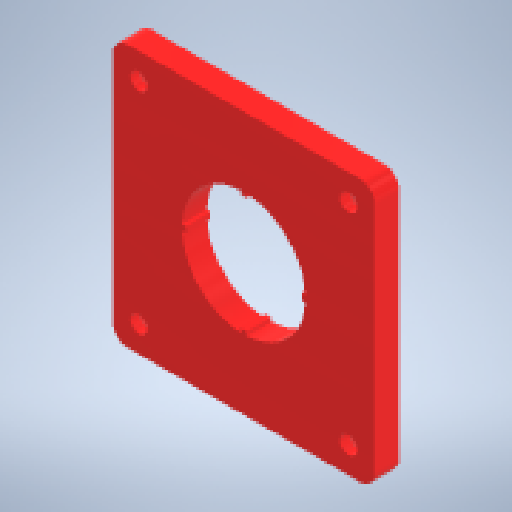
# Autodesk Inventor part: Parte1
Saved by Autodesk Inventor 2024 (Build 280153000, 153)
## iProperties
Created: 2023-12-16
Part Number: Parte1
Material: Generico
Document SubType Name: Modeling
Designer: cecca
Density: 1 g/cm^3
Appearance: Rosso chiaro
Author: cecca
Autodesk Inventor part; units mm, degrees
ref_plane "YZ Plane" through (0, 0, 0) normal (1, 0, 0) x (0, 1, 0)
ref_plane "XZ Plane" through (0, 0, 0) normal (0, 1, 0) x (-1, 0, 0)
ref_plane "XY Plane" through (0, 0, 0) normal (0, 0, 1) x (1, 0, 0)
sketch "Schizzo1" plane through (0, 0, 0) normal (0, 0, 1) x (1, 0, 0)
  line L0 (37.5, -42.5) -> (-37.5, -42.5)
  line L1 (-42.5, -37.5) -> (-42.5, 37.5)
  line L2 (-37.5, 42.5) -> (37.5, 42.5)
  line L3 (42.5, 37.5) -> (42.5, -37.5)
  line L4 (42.5, -42.5) -> (-42.5, 42.5) construction
  line L5 (-42.5, -42.5) -> (42.5, 42.5) construction
  arc A0 (-42.5, -37.5) -> (-37.5, -42.5) centre (-37.5, -37.5) ccw
  line L6 (-42.5, 42.5) -> (42.5, -42.5) construction
  arc A1 (-37.5, 42.5) -> (-42.5, 37.5) centre (-37.5, 37.5) ccw
  arc A2 (37.5, -42.5) -> (42.5, -37.5) centre (37.5, -37.5) ccw
  arc A3 (42.5, 37.5) -> (37.5, 42.5) centre (37.5, 37.5) ccw
  circle A4 centre (-34, -34) radius 5.2
  circle A5 centre (-34, 34) radius 5.2
  circle A6 centre (34, -34) radius 5.2
  circle A7 centre (34, 34) radius 5.2
  circle A8 centre (0, 0) radius 12
  circle A9 centre (0, 0) radius 20
  dimension "d12" = 85
  dimension "d17" = 10.4
  dimension "d18" = 24
  dimension "d19" = 40
  constraints: 14 end point, 10 centre point, 8 point on circle, 2 coincident, 2 midpoint, 2 parallel, 1 horizontal, 1 perpendicular
  measures "d12" distance of L4.end L5.end
  measures "d17" diameter of A4
  measures "d18" diameter of A8
  measures "d19" diameter of A9
extrude "Estrusione1" add sketch "Schizzo1" along normal mid plane 8 contours L0 A0 L1 A1 L2 A3 L3 A2
sketch "Schizzo2" plane through (0, 0, -4) normal (0, 0, -1) x (-1, 0, 0)
  circle A0 centre (-34, 34) radius 5.2 projected
  circle A1 centre (-34, 34) radius 5.2
  circle A2 centre (-34, 34) radius 2.5
  line L0 (-37.5, 42.5) -> (37.5, 42.5) projected
  line L1 (0, 42.5) -> (0, -42.5)
  line L2 (-37.5, -42.5) -> (37.5, -42.5) projected
  line L3 (-42.5, -37.5) -> (-42.5, 37.5) projected
  line L4 (-42.5, 0) -> (42.5, 0)
  line L5 (42.5, 37.5) -> (42.5, -37.5) projected
  circle A3 centre (34, 34) radius 5.2
  circle A4 centre (34, 34) radius 2.5
  circle A5 centre (-34, -34) radius 5.2
  circle A6 centre (-34, -34) radius 2.5
  circle A7 centre (34, -34) radius 2.5
  circle A8 centre (34, -34) radius 5.2
  point P0 (0, 0)
  dimension "d22" = 5
  constraints: 8 centre point, 6 symmetric about line, 4 end point, 4 midpoint, 2 coincident, 6 other
  measures "d22" diameter of A2
extrude "Estrusione2" add sketch "Schizzo2" against normal blind 8 contours A3
mirror "Speculare1" about plane through (0, 0, 0) normal (1, 0, 0) of "Estrusione2"
mirror "Speculare2" about plane through (0, 0, 0) normal (0, 1, 0) of "Estrusione2", "Speculare1"
sketch "Schizzo3" plane through (0, 0, -4) normal (0, 0, -1) x (-1, 0, 0)
  line L0 (37.5, -42.5) -> (-37.5, -42.5) projected
  line L1 (0, -42.5) -> (0, -40.5)
  line L2 (-37.5, -40.5) -> (37.5, -40.5)
  line L3 (-42.5, -37.5) -> (-42.5, 37.5) projected
  line L4 (-42.5, 0) -> (42.5, 0)
  line L5 (42.5, 37.5) -> (42.5, -37.5) projected
  line L6 (0, -42.5) -> (0, 42.5)
  line L7 (-37.5, 42.5) -> (37.5, 42.5) projected
  line L8 (-37.5, 40.5) -> (37.5, 40.5)
  line L9 (-42.5, 0) -> (-40.5, 0)
  line L10 (-40.5, -37.5) -> (-40.5, 37.5)
  line L11 (40.5, -37.5) -> (40.5, 37.5)
  arc A0 (37.5, -40.5) -> (40.5, -37.5) centre (37.5, -37.5) ccw
  arc A1 (-40.5, -37.5) -> (-37.5, -40.5) centre (-37.5, -37.5) ccw
  arc A2 (40.5, 37.5) -> (37.5, 40.5) centre (37.5, 37.5) ccw
  arc A3 (-37.5, 40.5) -> (-40.5, 37.5) centre (-37.5, 37.5) ccw
  circle A4 centre (0, 0) radius 20 projected
  circle A5 centre (0, 0) radius 25
  dimension "d25" = 2
  dimension "d27" = 2
  constraints: 16 end point, 8 point on circle, 7 symmetric about line, 5 centre point, 4 midpoint, 2 vertical, 1 coincident, 1 parallel, 1 point on line, 3 other
  measures "d25" distance of L1.start L1.end
  measures "d27" distance of L4.start L9.end
extrude "Estrusione3" cut sketch "Schizzo3" against normal blind 1 contours A1 L10 L4 A5 L6 L2 | L6 A5 L4 L11 A0 L2 | L10 A3 L8 L6 A5 L4 | A5 L6 L8 A2 L11 L4
sketch "Schizzo4" plane through (0, 0, -3) normal (0, 0, -1) x (-1, 0, 0)
  line L0 (37.5, -40.5) -> (-37.5, -40.5) projected
  line L1 (0, -40.5) -> (0, -38.5)
  line L2 (-37.5, -38.5) -> (37.5, -38.5)
  line L3 (-42.5, 37.5) -> (-42.5, -37.5) projected
  line L4 (-37.5, -42.5) -> (37.5, -42.5) projected
  line L5 (37.5, 42.5) -> (-37.5, 42.5) projected
  line L6 (-37.5, 38.5) -> (37.5, 38.5)
  line L7 (-38.4396, 0) -> (-0.9396, 0) construction
  line L8 (-40.5, -37.5) -> (-40.5, 37.5) projected
  line L9 (-40.5, 0) -> (-38.5, 0)
  line L10 (-38.5, -37.5) -> (-38.5, 37.5)
  arc A0 (-37.5, 38.5) -> (-38.5, 37.5) centre (-37.5, 37.5) ccw
  line L11 (38.5, -37.5) -> (38.5, 37.5)
  arc A1 (38.5, 37.5) -> (37.5, 38.5) centre (37.5, 37.5) ccw
  arc A2 (-38.5, -37.5) -> (-37.5, -38.5) centre (-37.5, -37.5) ccw
  arc A3 (37.5, -38.5) -> (38.5, -37.5) centre (37.5, -37.5) ccw
  point P0 (0, 0)
  dimension "d31" = 2
  dimension "d35" = 2
  dimension "d36" = 75
  constraints: 14 end point, 8 point on circle, 4 centre point, 2 midpoint, 2 parallel, 1 horizontal, 1 tangent, 1 vertical
  measures "d31" distance of L1.start L1.end
  measures "d35" distance of L9.start L9.end
  measures "d36" distance of L10.start L10.end
extrude "Estrusione4" cut sketch "Schizzo4" against normal blind 1.5 from surface at 0
sketch "Schizzo5" plane through (37.5, -38.5, -1.5) normal (0, 0, -1) x (-1, 0, 0)
  circle A0 centre (3.5, 4.5) radius 2.5 projected
  circle A1 centre (3.5, 4.5) radius 2.5
  point P0 (37.5, 38.5)
  constraints: 1 centre point, 1 coincident
hole "Foro1" at (34, -34, -1.5) direction (0, 0, 1) diameter 5.5 end through all countersink diameter 10.4 countersink angle 90 clearance for "Vite a testa svasata piana ISO 2009/7046" size "M5" standard "ISO"
mirror "Speculare3" about plane through (0, 0, 0) normal (1, 0, 0) of "Foro1"
mirror "Speculare4" about plane through (0, 0, 0) normal (0, 1, 0) of "Foro1", "Speculare3"
sketch "Schizzo6" plane through (31.3942, -38.5, -1.5) normal (0, 0, -1) x (-1, 0, 0)
  line L0 (62.7885, 0) -> (0, 0) projected
  line L1 (31.3942, 0) -> (31.3942, 3)
  line L2 (31.3942, 3) -> (57.3377, 3)
  line L3 (31.3942, 3) -> (5.4507, 3)
  line L4 (-7.1058, 1) -> (-7.1058, 76) projected
  line L5 (-7.1058, 38.5) -> (-4.1058, 38.5)
  line L6 (-4.1058, 38.5) -> (-4.1058, 64.4435)
  line L7 (-4.1058, 38.5) -> (-4.1058, 12.5565)
  line L8 (-11.1058, 1) -> (-11.1058, 76) projected
  line L9 (-11.1058, 38.5) -> (73.8942, 38.5)
  line L10 (73.8942, 76) -> (73.8942, 1) projected
  line L11 (31.3942, -3.9455) -> (31.3942, 81)
  line L12 (-6.1058, 81) -> (68.8942, 81) projected
  line L13 (31.3942, 74) -> (57.3377, 74)
  line L14 (31.3942, 74) -> (5.4507, 74)
  line L15 (66.8942, 38.5) -> (66.8942, 64.4435)
  line L16 (66.8942, 38.5) -> (66.8942, 12.5565)
  arc A0 (66.8942, 12.5565) -> (57.3377, 3) centre (66.8942, 3) ccw
  arc A1 (57.3377, 74) -> (66.8942, 64.4435) centre (66.8942, 74) ccw
  arc A2 (5.4507, 3) -> (-4.1058, 12.5565) centre (-4.1058, 3) ccw
  arc A3 (-4.1058, 64.4435) -> (5.4507, 74) centre (-4.1058, 74) ccw
  point P0 (31.3942, 38.5)
  dimension "d46" = 3
  dimension "d47" = 25.9435
  dimension "d48" = 25.9435
  dimension "d49" = 3
  dimension "d51" = 25.9435
  constraints: 24 end point, 8 point on circle, 8 symmetric about line, 5 midpoint, 4 centre point, 2 horizontal, 2 perpendicular, 2 vertical, 2 other
  measures "d46" distance of L1.start L1.end
  measures "d47" distance of L1.end L2.end
  measures "d48" distance of L3.end L1.end
  measures "d49" distance of L5.start L5.end
  measures "d51" distance of L7.end L5.end
extrude "Estrusione5" cut sketch "Schizzo6" against normal blind 1
sketch "Schizzo8" plane through (0, 0, -4) normal (0, 0, -1) x (-1, 0, 0)
  line L0 (-1, 21.321) -> (1, 21.321)
  line L1 (1, 21.321) -> (1, 18.679)
  line L2 (1, 18.679) -> (-1, 18.679)
  line L3 (-1, 18.679) -> (-1, 21.321)
  circle A0 centre (0, 0) radius 20 projected
  line L4 (-1, 21.321) -> (1, 18.679) construction
  line L5 (1, 21.321) -> (-1, 18.679) construction
  point P0 (0, 20)
  point P1 (1, 19.975)
  point P2 (-1, 19.975)
  dimension "d54" = 2
  dimension "d55" = 2.642
  constraints: 12 end point, 2 midpoint, 2 parallel, 1 horizontal, 1 perpendicular, 2 other
  measures "d54" distance of L1.end L2.end
  measures "d55" distance of L0.end L1.end
sketch "Schizzo9" plane through (0, 0, -3) normal (0, 0, 1) x (1, 0, 0)
  circle A0 centre (0, 0) radius 25
  circle A1 centre (0, 0) radius 20
  dimension "d56" = 50
  constraints: 2 centre point, 2 coincident
  measures "d56" diameter of A0
extrude "Estrusione6" add sketch "Schizzo9" along normal blind 2.7
extrude "Estrusione7" add sketch "Schizzo8" against normal blind 8 contours A0 L1 L2 L3 picked at (0.1112, 19.1184)
pattern_circular "Serie circolare1" count 4 over 360 about axis through (0, 0, 0) along (0, 0, 1) of "Estrusione7"
